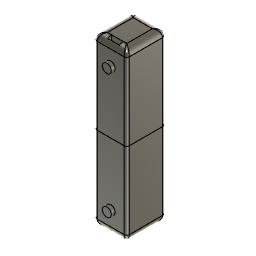
small leg (Autodesk Fusion 360 design; units mm, degrees)
Autodesk Fusion 360 part; units mm, degrees
sketch "Sketch1" plane through (0, 0, 0) normal (0, 0, 1) x (1, 0, 0)
  line L0 (25, 50) -> (55, 50)
  line L1 (55, 50) -> (55, 20)
  line L2 (55, 20) -> (25, 20)
  line L3 (25, 20) -> (25, 50)
  constraint horizontal L0
  constraint vertical L1
  constraint horizontal L2
  constraint vertical L3
extrude "Extrude1" add sketch "Sketch1" along normal blind 150 makes body 1
extrude "Extrude2" cut 1 faces at (55, 40, 50) along direction (-1, 0, 0) blind 5 on bodies 1 bodies 1
extrude "Extrude3" cut 1 faces at (33.3333, 30, 150) along direction (0, 0, -1) blind 10 on bodies 1 bodies 1
fillet "Fillet7" radius 5 1 faces at (33.3333, 30, 140) on bodies 1
fillet "Fillet8" radius 5 1 faces at (33.3333, 30, 0) on bodies 1
fillet "Fillet9" radius 2 14 faces at (33.3333, 50, 48.3333) (34.5665, 46.749, 0.3159) (35, 38.3333, 0) (34.9025, 24.4637, 0.0288) (41.6667, 20, 48.3333) (34.9025, 24.4637, 139.9712) (35, 38.3333, 140) (34.5665, 46.749, 139.6841) (29.4637, 31.5691, 139.9712) (25, 30, 48.3333) (29.4637, 31.5691, 0.0288) (46.749, 38.7668, 139.6841) (50, 40, 48.3333) (46.749, 38.7668, 0.3159) on bodies 1
sketch "Sketch4" plane through (0, 50, 0) normal (0, 1, 0) x (-1, 0, 0)
  line L0 (-48, 135) -> (-48, 5)
  line L1 (-48, 5) -> (-27, 5)
  line L2 (-27, 5) -> (-27, 135)
  line L3 (-27, 135) -> (-48, 135)
  line L4 (-37.5, 5) -> (-31, 5)
  line L5 (-31, 5) -> (-44, 5)
  line L6 (-44, 5) -> (-44, 38)
  line L7 (-44, 38) -> (-31, 38)
  line L8 (-31, 38) -> (-31, 5)
  line L9 (-31, 5) -> (-31, 10)
  line L10 (-31, 10) -> (-44, 10)
  line L11 (-44, 10) -> (-44, 33)
  line L12 (-44, 33) -> (-31, 33)
  line L13 (-31, 33) -> (-31, 10)
  circle A0 centre (-37.5, 16.5) radius 3.5
  line L14 (-44, 102) -> (-31, 102)
  line L15 (-44, 107) -> (-31, 107)
  line L16 (-31, 102) -> (-31, 135)
  line L17 (-44, 130) -> (-44, 107)
  line L18 (-44, 135) -> (-44, 102)
  line L19 (-31, 130) -> (-44, 130)
  line L20 (-31, 135) -> (-44, 135)
  circle A1 centre (-37.5, 123.5) radius 3.5
  constraint midpoint L1 L4.start
  constraint parallel L1 L4
  constraint horizontal L5
  constraint vertical L6
  constraint horizontal L7
  constraint vertical L8
  constraint perpendicular L4 L9
  constraint horizontal L10
  constraint vertical L11
  constraint horizontal L12
  constraint vertical L13
extrude "Extrude4" cut sketch "Sketch4" against normal blind 27 contours L6 L8 L10 L11 L12 L13 | A0 bodies 1
sketch "Sketch5" plane through (0, 0, 10) normal (0, 0, 1) x (-1, 0, 0)
  line L0 (-44, -50) -> (-31, -50)
  line L1 (-31, -50) -> (-31, -23)
  line L2 (-31, -23) -> (-44, -23)
  line L3 (-44, -23) -> (-44, -50)
  line L4 (-41.5185, -23) -> (-32.5185, -23)
  line L5 (-32.5185, -23) -> (-32.5185, -26)
  line L6 (-32.5185, -26) -> (-41.5185, -26)
  line L7 (-41.5185, -26) -> (-41.5185, -23)
  dimension "d42" = 9
  dimension "d43" = 3
  constraint horizontal L4
  constraint vertical L5
  constraint horizontal L6
  constraint vertical L7
  constraint coincident L2 L4.start
  measures "d42" distance of L4.start L4.end
  measures "d43" distance of L4.start L6.end
extrude "Extrude5" cut sketch "Sketch5" against normal blind 11 contours L2 L4 L5 L6 L7 bodies 1
extrude "Extrude6" add sketch "Sketch4" against normal blind 4 from surface at -30 contours A0 bodies 1
extrude "Extrude7" cut sketch "Sketch4" against normal blind 27 contours L15 L16 L17 L18 L19 | A1 bodies 1
extrude "Extrude8" add sketch "Sketch4" against normal blind 4 from surface at -30 contours A1 bodies 1
sketch "Sketch6" plane through (0, 0, 130) normal (0, 0, -1) x (1, 0, 0)
  line L0 (31, -50) -> (44, -50)
  line L1 (44, -50) -> (44, -23)
  line L2 (44, -23) -> (31, -23)
  line L3 (31, -23) -> (31, -50)
  line L4 (41.5626, -23) -> (32.5626, -23)
  line L5 (32.5626, -23) -> (32.5626, -26)
  line L6 (32.5626, -26) -> (41.5626, -26)
  line L7 (41.5626, -26) -> (41.5626, -23)
  dimension "d54" = 9
  dimension "d55" = 3
  constraint horizontal L4
  constraint vertical L5
  constraint horizontal L6
  constraint vertical L7
  constraint coincident L2 L4.start
  measures "d54" distance of L4.start L4.end
  measures "d55" distance of L4.start L6.end
extrude "Extrude14" cut 1 faces at (35.3333, 23, 114.6667) along direction (0, -1, 0) blind 1 on bodies 1 bodies 1
extrude "Extrude15" cut 1 faces at (37.2404, 16, 122.3626) along direction (0, 1, 0) blind 1 on bodies 1 bodies 1
extrude "Extrude16" cut 1 faces at (37.1409, 16, 17.4466) along direction (0, 1, 0) blind 1 on bodies 1 bodies 1
extrude "Extrude17" cut 1 faces at (37.2404, 17, 122.3626) along direction (0, 1, 0) blind 1 on bodies 1 bodies 1
extrude "Extrude18" cut sketch "Sketch4" against normal blind 9 contours L3 L16 L18 L19 L20 | L1 L4 L5 L6 L8 L9 L10 | L14 L15 L16 L18 | L6 L7 L8 L12 bodies 1
extrude "Extrude19" cut 2 faces at (39.6667, 41, 131.6667) (39.6667, 41, 105.3333) along direction (0, -1, 0) blind 1 on bodies 1 bodies 1
sketch "Sketch7" plane through (0, 0, 130) normal (0, 0, -1) x (1, 0, 0)
  line L0 (31, -40) -> (44, -40)
  line L1 (44, -40) -> (44, -22)
  line L2 (44, -22) -> (31, -22)
  line L3 (31, -22) -> (31, -40)
  line L4 (42.2889, -22) -> (33.2889, -22)
  line L5 (33.2889, -22) -> (33.2889, -25)
  line L6 (33.2889, -25) -> (42.2889, -25)
  line L7 (42.2889, -25) -> (42.2889, -22)
  dimension "d78" = 9
  dimension "d79" = 3
  constraint horizontal L4
  constraint vertical L5
  constraint horizontal L6
  constraint vertical L7
  constraint coincident L2 L4.start
  measures "d78" distance of L4.start L4.end
  measures "d79" distance of L4.start L6.end
extrude "Extrude20" cut sketch "Sketch7" against normal blind 18 contours L2 L4 L5 L6 L7 bodies 1
extrude "Extrude21" add 1 faces at (37.2404, 18, 122.3626) along direction (0, -1, 0) blind 1 on bodies 1 bodies 1
sketch "Sketch8" plane through (50, 0, 0) normal (1, 0, 0) x (0, 1, 0)
  line L0 (22, 135) -> (22, 5)
  line L1 (22, 5) -> (48, 5)
  line L2 (48, 5) -> (48, 135)
  line L3 (48, 135) -> (22, 135)
  line L4 (48, 70) -> (22, 70)
  line L5 (48, 75) -> (22, 75)
  line L6 (48, 65) -> (22, 65)
  line L7 (22, 75) -> (48, 75)
  line L8 (48, 65) -> (22, 65)
  constraint midpoint L2 L4.start
  constraint midpoint L0 L4.end
extrude "Extrude22" cut sketch "Sketch8" against normal blind 40 contours L0 L2 L4 L5 L7 | L0 L2 L4 L6 L8 bodies 1
extrude "Extrude23" cut 1 faces at (41.6667, 48, 68.3333) along direction (0, 1, 0) blind 5 on bodies 1 bodies 1
extrude "Extrude24" cut 1 faces at (41.6667, 22, 71.6667) along direction (0, -1, 0) blind 16 on bodies 1 bodies 1 makes body 2 at (25, 30.6667, 25)
copy_body "Body->Comp1" bodies 1 removing the originals makes body 3 in component "Component"
copy_body "Body->Comp2" bodies 2 removing the originals makes body 4 in component "Component'"
extrude "Extrude9" [suppressed]
extrude "Extrude10" [suppressed]
extrude "Extrude11" [suppressed]
extrude "Extrude12" [suppressed]
extrude "Extrude13" [suppressed]
fillet "Fillet4" [suppressed]
fillet "Fillet5" [suppressed]
fillet "Fillet6" [suppressed]
sketch "Sketch3" plane through (0, 50, 0) normal (0, 1, 0) x (-1, 0, 0)
  line L0 (-48, 140) -> (-48, 5)
  line L1 (-48, 5) -> (-27, 5)
  line L2 (-27, 5) -> (-27, 140)
  line L3 (-27, 140) -> (-48, 140)
  line L4 (-44.5, 5) -> (-30.5, 5)
  line L5 (-30.5, 5) -> (-30.5, 30)
  line L6 (-30.5, 30) -> (-44.5, 30)
  line L7 (-44.5, 30) -> (-44.5, 5)
  constraint horizontal L4
  constraint vertical L5
  constraint horizontal L6
  constraint vertical L7
fillet "Fillet1" [suppressed]
fillet "Fillet2" [suppressed]
fillet "Fillet3" [suppressed]
component "Component" placed x (1, 0, 0) y (0, 1, 0) z (0, 0, 1) at (0, 0, -10)
component "Component'" placed x (1, 0, 0) y (0, 1, 0) z (0, 0, 1) at (0, 0, 0)
